Autodesk Inventor part; units mm, degrees
(part 2 of 2)
sketch "Sketch5" plane through (-0.0003, -144.9621, -142.4319) normal (0, 0, -1) x (-1, 0, 0)
  line L0 (-2.9666, 137.688) -> (-2.1497, 137.688)
  line L1 (-2.1497, 137.688) -> (-2.1497, 133.7853)
  line L2 (-2.1497, 133.7853) -> (-2.9666, 133.7853)
  line L3 (-2.9666, 133.7853) -> (-2.9666, 135.2375)
  line L4 (-2.9666, 135.2375) -> (-8.328, 135.2375)
  line L5 (-8.328, 135.2375) -> (-8.328, 133.7853)
  line L6 (-8.328, 133.7853) -> (-9.0606, 133.7853)
  spline S0 degree 2 poles (-9.0606, 133.7853) (-9.0606, 134.6086) (-9.5274, 135.3866) (-10.1757, 135.4385) knots 0 0 0 1 2 2 2
  line L7 (-10.1757, 135.4385) -> (-10.1757, 136.2683)
  line L8 (-10.1757, 136.2683) -> (-2.9666, 136.2683)
  line L9 (-2.9666, 136.2683) -> (-2.9666, 137.688)
  spline S1 degree 2 poles (-8.9569, 129.9474) (-9.106, 129.7205) (-9.2291, 129.1175) (-9.2291, 128.6767) knots 0 0 0 1 2 2 2
  line L10 (-9.2291, 128.6767) -> (-9.2291, 127.62)
  line L11 (-9.2291, 127.62) -> (-6.221, 127.62)
  line L12 (-6.221, 127.62) -> (-6.221, 128.5535)
  spline S2 degree 2 poles (-6.221, 128.5535) (-6.221, 129.0138) (-6.3831, 129.7464) (-6.636, 129.9992) knots 0 0 0 1 2 2 2
  spline S3 degree 2 poles (-6.636, 129.9992) (-6.8564, 130.2326) (-7.4787, 130.453) (-7.8937, 130.453) knots 0 0 0 1 2 2 2
  spline S4 degree 2 poles (-7.8937, 130.453) (-8.2437, 130.453) (-8.7818, 130.2067) (-8.9569, 129.9474) knots 0 0 0 1 2 2 2
  line L13 (-5.6311, 129.902) -> (-2.1497, 132.748)
  line L14 (-2.1497, 132.748) -> (-2.1497, 131.3671)
  line L15 (-2.1497, 131.3671) -> (-5.3329, 128.8388)
  line L16 (-5.3329, 128.8388) -> (-5.3329, 127.62)
  line L17 (-5.3329, 127.62) -> (-2.1497, 127.62)
  line L18 (-2.1497, 127.62) -> (-2.1497, 126.5568)
  line L19 (-2.1497, 126.5568) -> (-10.1497, 126.5568)
  line L20 (-10.1497, 126.5568) -> (-10.1497, 128.6184)
  spline S5 degree 2 poles (-10.1497, 128.6184) (-10.1497, 129.3056) (-10.0006, 130.2326) (-9.7283, 130.654) knots 0 0 0 1 2 2 2
  spline S6 degree 2 poles (-9.7283, 130.654) (-9.4561, 131.0754) (-8.6068, 131.5616) (-7.9779, 131.5616) knots 0 0 0 1 2 2 2
  spline S7 degree 2 poles (-7.9779, 131.5616) (-7.1027, 131.5616) (-5.9163, 130.667) (-5.6311, 129.902) knots 0 0 0 1 2 2 2
  circle A0 centre (-58.0001, 28.9999) radius 15
  circle A1 centre (-58.0001, 28.9999) radius 17.5
  circle A2 centre (-58.0002, 115.962) radius 15
  circle A3 centre (-58.0002, 115.962) radius 17.5
  spline S8 degree 2 poles (-53.3136, 62.2242) (-52.7949, 62.2242) (-52.017, 61.9487) (-51.7414, 61.6569) knots 0 0 0 1 2 2 2
  spline S9 degree 2 poles (-51.7414, 61.6569) (-51.4254, 61.3409) (-51.2228, 60.4252) (-51.2228, 59.8498) knots 0 0 0 1 2 2 2
  line L21 (-51.2228, 59.8498) -> (-51.2228, 58.6829)
  line L22 (-51.2228, 58.6829) -> (-54.9829, 58.6829)
  line L23 (-54.9829, 58.6829) -> (-54.9829, 60.0038)
  spline S10 degree 2 poles (-54.9829, 60.0038) (-54.9829, 60.5548) (-54.829, 61.3085) (-54.6426, 61.5921) knots 0 0 0 1 2 2 2
  spline S11 degree 2 poles (-54.6426, 61.5921) (-54.4238, 61.9163) (-53.7512, 62.2242) (-53.3136, 62.2242) knots 0 0 0 1 2 2 2
  spline S12 degree 2 poles (-55.6069, 62.4754) (-55.9473, 61.9487) (-56.1337, 60.7898) (-56.1337, 59.9308) knots 0 0 0 1 2 2 2
  line L24 (-56.1337, 59.9308) -> (-56.1337, 57.3539)
  line L25 (-56.1337, 57.3539) -> (-46.1337, 57.3539)
  line L26 (-46.1337, 57.3539) -> (-46.1337, 58.6829)
  line L27 (-46.1337, 58.6829) -> (-50.1126, 58.6829)
  line L28 (-50.1126, 58.6829) -> (-50.1126, 60.2064)
  line L29 (-50.1126, 60.2064) -> (-46.1337, 63.3668)
  line L30 (-46.1337, 63.3668) -> (-46.1337, 65.0929)
  line L31 (-46.1337, 65.0929) -> (-50.4854, 61.5354)
  spline S13 degree 2 poles (-50.4854, 61.5354) (-50.8419, 62.4916) (-52.3249, 63.6099) (-53.4189, 63.6099) knots 0 0 0 1 2 2 2
  spline S14 degree 2 poles (-53.4189, 63.6099) (-54.205, 63.6099) (-55.2666, 63.0022) (-55.6069, 62.4754) knots 0 0 0 1 2 2 2
  spline S15 degree 2 poles (-38.2398, 60.268) (-36.6644, 60.268) (-34.9918, 58.952) (-34.9918, 57.8434) knots 0 0 0 1 2 2 2
  spline S16 degree 2 poles (-34.9918, 57.8434) (-34.9918, 56.7348) (-36.6644, 55.4122) (-38.2398, 55.4122) knots 0 0 0 1 2 2 2
  spline S17 degree 2 poles (-38.2398, 55.4122) (-39.0177, 55.4122) (-40.2495, 55.7494) (-40.6579, 56.067) knots 0 0 0 1 2 2 2
  spline S18 degree 2 poles (-40.6579, 56.067) (-41.0858, 56.3977) (-41.4878, 57.2664) (-41.4878, 57.8434) knots 0 0 0 1 2 2 2
  spline S19 degree 2 poles (-41.4878, 57.8434) (-41.4878, 58.4009) (-41.0728, 59.2956) (-40.6579, 59.6132) knots 0 0 0 1 2 2 2
  spline S20 degree 2 poles (-40.6579, 59.6132) (-40.256, 59.9244) (-39.0307, 60.268) (-38.2398, 60.268) knots 0 0 0 1 2 2 2
  spline S21 degree 2 poles (-38.2398, 54.3037) (-37.2544, 54.3037) (-35.692, 54.7964) (-35.1604, 55.2567) knots 0 0 0 1 2 2 2
  spline S22 degree 2 poles (-35.1604, 55.2567) (-34.6223, 55.7299) (-34.0712, 57.0265) (-34.0712, 57.8369) knots 0 0 0 1 2 2 2
  spline S23 degree 2 poles (-34.0712, 57.8369) (-34.0712, 58.6213) (-34.6028, 59.9244) (-35.1604, 60.4171) knots 0 0 0 1 2 2 2
  spline S24 degree 2 poles (-35.1604, 60.4171) (-35.692, 60.8839) (-37.2673, 61.3766) (-38.2398, 61.3766) knots 0 0 0 1 2 2 2
  spline S25 degree 2 poles (-38.2398, 61.3766) (-39.2382, 61.3766) (-40.7941, 60.8709) (-41.3257, 60.4171) knots 0 0 0 1 2 2 2
  spline S26 degree 2 poles (-41.3257, 60.4171) (-41.8378, 59.9633) (-42.4083, 58.6537) (-42.4083, 57.8369) knots 0 0 0 1 2 2 2
  spline S27 degree 2 poles (-42.4083, 57.8369) (-42.4083, 57.033) (-41.8573, 55.7299) (-41.3257, 55.2631) knots 0 0 0 1 2 2 2
  spline S28 degree 2 poles (-41.3257, 55.2631) (-40.7746, 54.8028) (-39.2446, 54.3037) (-38.2398, 54.3037) knots 0 0 0 1 2 2 2
  line L32 (-35.1863, 82.7186) -> (-38.1555, 82.7186)
  line L33 (-38.1555, 82.7186) -> (-38.1555, 86.3944)
  line L34 (-38.1555, 86.3944) -> (-39.102, 86.3944)
  line L35 (-39.102, 86.3944) -> (-39.102, 82.7186)
  line L36 (-39.102, 82.7186) -> (-41.2933, 82.7186)
  line L37 (-41.2933, 82.7186) -> (-41.2933, 86.6602)
  line L38 (-41.2933, 86.6602) -> (-42.2398, 86.6602)
  line L39 (-42.2398, 86.6602) -> (-42.2398, 81.6554)
  line L40 (-42.2398, 81.6554) -> (-34.2398, 81.6554)
  line L41 (-34.2398, 81.6554) -> (-34.2398, 86.6602)
  line L42 (-34.2398, 86.6602) -> (-35.1863, 86.6602)
  line L43 (-35.1863, 86.6602) -> (-35.1863, 82.7186)
  line L44 (-42.2398, 77.2469) -> (-42.2398, 76.1837)
  line L45 (-42.2398, 76.1837) -> (-34.2398, 76.1837)
  line L46 (-34.2398, 76.1837) -> (-34.2398, 80.8191)
  line L47 (-34.2398, 80.8191) -> (-35.1863, 80.8191)
  line L48 (-35.1863, 80.8191) -> (-35.1863, 77.2469)
  line L49 (-35.1863, 77.2469) -> (-42.2398, 77.2469)
  spline S29 degree 2 poles (-25.1959, 17.9986) (-24.6221, 17.9986) (-23.7761, 17.6777) (-23.4163, 17.3179) knots 0 0 0 1 2 2 2
  spline S30 degree 2 poles (-23.4163, 17.3179) (-23.0079, 16.9289) (-22.6967, 15.7328) (-22.6967, 14.7604) knots 0 0 0 1 2 2 2
  line L50 (-22.6967, 14.7604) -> (-22.6967, 13.6712)
  line L51 (-22.6967, 13.6712) -> (-27.4811, 13.6712)
  line L52 (-27.4811, 13.6712) -> (-27.4811, 14.9938)
  spline S31 degree 2 poles (-27.4811, 14.9938) (-27.4811, 15.7425) (-27.2769, 16.7539) (-27.0241, 17.1331) knots 0 0 0 1 2 2 2
  spline S32 degree 2 poles (-27.0241, 17.1331) (-26.7323, 17.5707) (-25.8182, 17.9986) (-25.1959, 17.9986) knots 0 0 0 1 2 2 2
  line L53 (-28.862, 12.0764) -> (-16.862, 12.0764)
  line L54 (-16.862, 12.0764) -> (-16.862, 13.6712)
  line L55 (-16.862, 13.6712) -> (-21.3352, 13.6712)
  line L56 (-21.3352, 13.6712) -> (-21.3352, 15.0229)
  spline S33 degree 2 poles (-21.3352, 15.0229) (-21.3352, 16.3066) (-21.9673, 17.9889) (-22.58, 18.6113) knots 0 0 0 1 2 2 2
  spline S34 degree 2 poles (-22.58, 18.6113) (-23.0662, 19.1072) (-24.4665, 19.6615) (-25.2445, 19.6615) knots 0 0 0 1 2 2 2
  spline S35 degree 2 poles (-25.2445, 19.6615) (-26.2461, 19.6615) (-27.6561, 18.903) (-28.1132, 18.232) knots 0 0 0 1 2 2 2
  spline S36 degree 2 poles (-28.1132, 18.232) (-28.5119, 17.6583) (-28.862, 16.1607) (-28.862, 15.091) knots 0 0 0 1 2 2 2
  line L57 (-28.862, 15.091) -> (-28.862, 12.0764)
  line L58 (-10.1757, 136.2683) -> (-10.1757, 135.4385)
  spline S37 degree 2 poles (-10.1757, 135.4385) (-9.5274, 135.3866) (-9.0606, 134.6086) (-9.0606, 133.7853) knots 0 0 0 1 2 2 2
  line L59 (-9.0606, 133.7853) -> (-8.328, 133.7853)
  line L60 (-8.328, 133.7853) -> (-8.328, 135.2375)
  line L61 (-8.328, 135.2375) -> (-2.9666, 135.2375)
  line L62 (-2.9666, 135.2375) -> (-2.9666, 133.7853)
  line L63 (-2.9666, 133.7853) -> (-2.1497, 133.7853)
  line L64 (-2.1497, 133.7853) -> (-2.1497, 137.688)
  line L65 (-2.1497, 137.688) -> (-2.9666, 137.688)
  line L66 (-2.9666, 137.688) -> (-2.9666, 136.2683)
  line L67 (-2.9666, 136.2683) -> (-10.1757, 136.2683)
  line L68 (-46.0033, 82.349) -> (-46.0033, 83.678)
  line L69 (-46.0033, 83.678) -> (-50.8169, 83.678)
  line L70 (-50.8169, 83.678) -> (-50.8169, 88.135)
  line L71 (-50.8169, 88.135) -> (-52, 88.135)
  line L72 (-52, 88.135) -> (-52, 83.678)
  line L73 (-52, 83.678) -> (-54.8201, 83.678)
  line L74 (-54.8201, 83.678) -> (-54.8201, 88.3295)
  line L75 (-54.8201, 88.3295) -> (-56.0033, 88.3295)
  line L76 (-56.0033, 88.3295) -> (-56.0033, 82.349)
  line L77 (-56.0033, 82.349) -> (-46.0033, 82.349)
  line L78 (-42.2398, 68.2356) -> (-42.2398, 67.1724)
  line L79 (-42.2398, 67.1724) -> (-37.222, 67.1724)
  spline S38 degree 2 poles (-37.222, 67.1724) (-36.6839, 67.1724) (-35.9383, 67.0298) (-35.6336, 66.8288) knots 0 0 0 1 2 2 2
  spline S39 degree 2 poles (-35.6336, 66.8288) (-35.3095, 66.6148) (-34.9788, 65.8369) (-34.9788, 65.3377) knots 0 0 0 1 2 2 2
  spline S40 degree 2 poles (-34.9788, 65.3377) (-34.9788, 64.8061) (-35.3095, 64.067) (-35.6336, 63.8531) knots 0 0 0 1 2 2 2
  spline S41 degree 2 poles (-35.6336, 63.8531) (-35.9383, 63.6521) (-36.6904, 63.5095) (-37.2479, 63.5095) knots 0 0 0 1 2 2 2
  line L80 (-37.2479, 63.5095) -> (-42.2398, 63.5095)
  line L81 (-42.2398, 63.5095) -> (-42.2398, 62.4463)
  line L82 (-42.2398, 62.4463) -> (-37.2479, 62.4463)
  spline S42 degree 2 poles (-37.2479, 62.4463) (-36.3921, 62.4463) (-35.2252, 62.7899) (-34.8103, 63.2113) knots 0 0 0 1 2 2 2
  spline S43 degree 2 poles (-34.8103, 63.2113) (-34.4408, 63.5808) (-34.0712, 64.631) (-34.0712, 65.3377) knots 0 0 0 1 2 2 2
  spline S44 degree 2 poles (-34.0712, 65.3377) (-34.0712, 66.0768) (-34.4343, 67.0881) (-34.8103, 67.4706) knots 0 0 0 1 2 2 2
  spline S45 degree 2 poles (-34.8103, 67.4706) (-35.2187, 67.8985) (-36.4116, 68.2356) (-37.2479, 68.2356) knots 0 0 0 1 2 2 2
  line L83 (-37.2479, 68.2356) -> (-42.2398, 68.2356)
  line L84 (-41.2933, 93.4414) -> (-42.2398, 93.4414)
  line L85 (-42.2398, 93.4414) -> (-42.2398, 87.0103)
  line L86 (-42.2398, 87.0103) -> (-41.2933, 87.0103)
  line L87 (-41.2933, 87.0103) -> (-41.2933, 89.6943)
  line L88 (-41.2933, 89.6943) -> (-34.2398, 89.6943)
  line L89 (-34.2398, 89.6943) -> (-34.2398, 90.7575)
  line L90 (-34.2398, 90.7575) -> (-41.2933, 90.7575)
  line L91 (-41.2933, 90.7575) -> (-41.2933, 93.4414)
  line L92 (-41.2933, 75.3733) -> (-42.2398, 75.3733)
  line L93 (-42.2398, 75.3733) -> (-42.2398, 68.9422)
  line L94 (-42.2398, 68.9422) -> (-41.2933, 68.9422)
  line L95 (-41.2933, 68.9422) -> (-41.2933, 71.6262)
  line L96 (-41.2933, 71.6262) -> (-34.2398, 71.6262)
  line L97 (-34.2398, 71.6262) -> (-34.2398, 72.6894)
  line L98 (-34.2398, 72.6894) -> (-41.2933, 72.6894)
  line L99 (-41.2933, 72.6894) -> (-41.2933, 75.3733)
  line L100 (-19.5848, 29.5999) -> (-19.5848, 29.4832)
  spline S46 degree 2 poles (-19.5848, 29.4832) (-19.4001, 29.2985) (-18.8749, 28.6469) (-18.6221, 28.2093) knots 0 0 0 1 2 2 2
  spline S47 degree 2 poles (-18.6221, 28.2093) (-18.3693, 27.7523) (-18.0289, 26.5756) (-18.0289, 25.8852) knots 0 0 0 1 2 2 2
  spline S48 degree 2 poles (-18.0289, 25.8852) (-18.0289, 25.1267) (-18.6318, 23.775) (-19.225, 23.2693) knots 0 0 0 1 2 2 2
  spline S49 degree 2 poles (-19.225, 23.2693) (-19.8377, 22.7539) (-21.6173, 22.1607) (-22.8523, 22.1607) knots 0 0 0 1 2 2 2
  spline S50 degree 2 poles (-22.8523, 22.1607) (-24.0095, 22.1607) (-25.8668, 22.7247) (-26.4795, 23.2304) knots 0 0 0 1 2 2 2
  spline S51 degree 2 poles (-26.4795, 23.2304) (-27.0824, 23.7458) (-27.7145, 25.1169) (-27.7145, 25.8852) knots 0 0 0 1 2 2 2
  spline S52 degree 2 poles (-27.7145, 25.8852) (-27.7145, 26.5853) (-27.3936, 27.6647) (-27.1408, 28.1218) knots 0 0 0 1 2 2 2
  spline S53 degree 2 poles (-27.1408, 28.1218) (-26.8782, 28.5983) (-26.3336, 29.2596) (-26.1391, 29.4735) knots 0 0 0 1 2 2 2
  line L101 (-26.1391, 29.4735) -> (-26.1391, 29.5999)
  line L102 (-26.1391, 29.5999) -> (-28.0646, 29.5999)
  spline S54 degree 2 poles (-28.0646, 29.5999) (-28.2785, 29.2012) (-28.6383, 28.3941) (-28.7647, 28.0051) knots 0 0 0 1 2 2 2
  spline S55 degree 2 poles (-28.7647, 28.0051) (-28.9009, 27.5578) (-29.0759, 26.4978) (-29.0759, 25.8949) knots 0 0 0 1 2 2 2
  spline S56 degree 2 poles (-29.0759, 25.8949) (-29.0759, 24.6793) (-28.2299, 22.715) (-27.4228, 21.9954) knots 0 0 0 1 2 2 2
  spline S57 degree 2 poles (-27.4228, 21.9954) (-26.5962, 21.266) (-24.3596, 20.4978) (-22.8523, 20.4978) knots 0 0 0 1 2 2 2
  spline S58 degree 2 poles (-22.8523, 20.4978) (-21.3352, 20.4978) (-19.0014, 21.2855) (-18.2234, 22.0051) knots 0 0 0 1 2 2 2
  spline S59 degree 2 poles (-18.2234, 22.0051) (-17.4357, 22.7247) (-16.648, 24.6988) (-16.648, 25.8657) knots 0 0 0 1 2 2 2
  spline S60 degree 2 poles (-16.648, 25.8657) (-16.648, 26.5853) (-16.8231, 27.48) (-16.9981, 28.0051) knots 0 0 0 1 2 2 2
  spline S61 degree 2 poles (-16.9981, 28.0051) (-17.1537, 28.501) (-17.4941, 29.2012) (-17.6788, 29.5999) knots 0 0 0 1 2 2 2
  line L103 (-17.6788, 29.5999) -> (-19.5848, 29.5999)
  spline S62 degree 2 poles (-7.8937, 130.453) (-7.4787, 130.453) (-6.8564, 130.2326) (-6.636, 129.9992) knots 0 0 0 1 2 2 2
  spline S63 degree 2 poles (-6.636, 129.9992) (-6.3831, 129.7464) (-6.221, 129.0138) (-6.221, 128.5535) knots 0 0 0 1 2 2 2
  line L104 (-6.221, 128.5535) -> (-6.221, 127.62)
  line L105 (-6.221, 127.62) -> (-9.2291, 127.62)
  line L106 (-9.2291, 127.62) -> (-9.2291, 128.6767)
  spline S64 degree 2 poles (-9.2291, 128.6767) (-9.2291, 129.1175) (-9.106, 129.7205) (-8.9569, 129.9474) knots 0 0 0 1 2 2 2
  spline S65 degree 2 poles (-8.9569, 129.9474) (-8.7818, 130.2067) (-8.2437, 130.453) (-7.8937, 130.453) knots 0 0 0 1 2 2 2
  spline S66 degree 2 poles (-9.7283, 130.654) (-10.0006, 130.2326) (-10.1497, 129.3056) (-10.1497, 128.6184) knots 0 0 0 1 2 2 2
  line L107 (-10.1497, 128.6184) -> (-10.1497, 126.5568)
  line L108 (-10.1497, 126.5568) -> (-2.1497, 126.5568)
  line L109 (-2.1497, 126.5568) -> (-2.1497, 127.62)
  line L110 (-2.1497, 127.62) -> (-5.3329, 127.62)
  line L111 (-5.3329, 127.62) -> (-5.3329, 128.8388)
  line L112 (-5.3329, 128.8388) -> (-2.1497, 131.3671)
  line L113 (-2.1497, 131.3671) -> (-2.1497, 132.748)
  line L114 (-2.1497, 132.748) -> (-5.6311, 129.902)
  spline S67 degree 2 poles (-5.6311, 129.902) (-5.9163, 130.667) (-7.1027, 131.5616) (-7.9779, 131.5616) knots 0 0 0 1 2 2 2
  spline S68 degree 2 poles (-7.9779, 131.5616) (-8.6068, 131.5616) (-9.4561, 131.0754) (-9.7283, 130.654) knots 0 0 0 1 2 2 2
  line L115 (-80, 1.9999) -> (3, 2)
  line L116 (2.9997, 142.9621) -> (3, 2)
  line L117 (2.9997, 142.9621) -> (-80.0003, 142.9619)
  line L118 (-80, 1.9999) -> (-80.0003, 142.9619)
  circle A4 centre (-65.2412, 59.9999) radius 3.35
  circle A5 centre (-65.2412, 84.962) radius 3.35
  line L119 (-14.0356, 12.0349) -> (-4.0356, 12.0349)
  line L120 (-4.0356, 12.0349) -> (-4.0357, 29.0349)
  line L121 (-4.0357, 29.0349) -> (-14.0357, 29.0349)
  line L122 (-14.0357, 29.0349) -> (-14.0356, 12.0349)
  line L123 (-63.526, 17.7389) -> (-63.526, 41.2748) construction
  line L124 (-63.526, 41.2748) -> (-53.9143, 41.2748) construction
  line L125 (-53.9143, 41.2748) -> (-53.9143, 17.7389) construction
  line L126 (-53.9143, 17.7389) -> (-63.526, 17.7389) construction
  line L127 (-63.308, 105.7482) -> (-63.308, 126.3521) construction
  line L128 (-63.308, 126.3521) -> (-53.7172, 126.3521) construction
  line L129 (-53.7172, 126.3521) -> (-53.7172, 105.7482) construction
  line L130 (-53.7172, 105.7482) -> (-63.308, 105.7482) construction
  spline S69 degree 2 poles (-57.7913, 18.1574) (-59.5954, 18.1574) (-60.4666, 19.1657) knots 0 0 0 1 1 1
  spline S70 degree 2 poles (-60.4666, 19.1657) (-61.1937, 20.0026) (-61.1937, 21.2099) knots 0 0 0 1 1 1
  spline S71 degree 2 poles (-61.1937, 21.2099) (-61.1937, 22.5545) (-59.4308, 24.2625) (-57.8805, 24.2625) knots 0 0 0 1 2 2 2
  spline S72 degree 2 poles (-57.8805, 24.2625) (-56.6251, 24.2625) (-55.1777, 23.508) (-54.382, 22.0674) (-54.382, 21.2099) knots 0 0 0 1 2 3 3 3
  spline S73 degree 2 poles (-54.382, 21.2099) (-54.382, 19.8449) (-56.1381, 18.1574) (-57.7913, 18.1574) knots 0 0 0 1 2 2 2
  spline S74 degree 2 poles (-57.7844, 19.2961) (-56.536, 19.2961) (-55.2875, 20.3868) (-55.2875, 21.2099) knots 0 0 0 1 2 2 2
  spline S75 degree 2 poles (-55.2875, 21.2099) (-55.2875, 22.0331) (-56.5428, 23.1238) (-57.8256, 23.1238) knots 0 0 0 1 2 2 2
  spline S76 degree 2 poles (-57.8256, 23.1238) (-59.0329, 23.1238) (-60.2814, 22.0263) (-60.2814, 21.2099) knots 0 0 0 1 2 2 2
  spline S77 degree 2 poles (-60.2814, 21.2099) (-60.2814, 20.3868) (-59.0398, 19.2961) (-57.7844, 19.2961) knots 0 0 0 1 2 2 2
  line L131 (-56.4742, 25.1131) -> (-56.6457, 26.2038)
  spline S78 degree 2 poles (-56.6457, 26.2038) (-55.9872, 26.293) (-55.2875, 27.1368) (-55.2875, 27.8982) knots 0 0 0 1 2 2 2
  spline S79 degree 2 poles (-55.2875, 27.8982) (-55.2875, 28.6596) (-55.9117, 29.4005) (-56.3302, 29.4005) knots 0 0 0 1 2 2 2
  spline S80 degree 2 poles (-56.3302, 29.4005) (-56.7006, 29.4005) (-56.9201, 29.0712) knots 0 0 0 1 1 1
  spline S81 degree 2 poles (-56.9201, 29.0712) (-57.0642, 28.8448) (-57.2905, 27.9394) knots 0 0 0 1 1 1
  spline S82 degree 2 poles (-57.2905, 27.9394) (-57.5992, 26.7252) (-58.0451, 25.7854) (-58.8408, 25.2984) (-59.3142, 25.2984) knots 0 0 0 1 2 3 3 3
  spline S83 degree 2 poles (-59.3142, 25.2984) (-59.7532, 25.2984) (-60.494, 25.6962) (-60.741, 26.0392) knots 0 0 0 1 2 2 2
  spline S84 degree 2 poles (-60.741, 26.0392) (-60.9331, 26.2999) (-61.1937, 27.1916) (-61.1937, 27.7061) knots 0 0 0 1 2 2 2
  spline S85 degree 2 poles (-61.1937, 27.7061) (-61.1937, 28.4744) (-60.7478, 29.6337) (-59.9933, 30.1894) (-59.3622, 30.2923) knots 0 0 0 1 2 3 3 3
  line L132 (-59.3622, 30.2923) -> (-59.2181, 29.2084)
  spline S86 degree 2 poles (-59.2181, 29.2084) (-59.7257, 29.133) (-60.2882, 28.4264) (-60.2882, 27.7816) knots 0 0 0 1 2 2 2
  spline S87 degree 2 poles (-60.2882, 27.7816) (-60.2882, 27.0202) (-59.7806, 26.3685) (-59.4445, 26.3685) knots 0 0 0 1 2 2 2
  spline S88 degree 2 poles (-59.4445, 26.3685) (-59.2318, 26.3685) (-59.0603, 26.5057) knots 0 0 0 1 1 1
  spline S89 degree 2 poles (-59.0603, 26.5057) (-58.882, 26.636) (-58.7654, 26.931) knots 0 0 0 1 1 1
  spline S90 degree 2 poles (-58.7654, 26.931) (-58.7036, 27.0956) (-58.4773, 27.9051) knots 0 0 0 1 1 1
  spline S91 degree 2 poles (-58.4773, 27.9051) (-58.1686, 29.0781) (-57.7707, 30.011) (-57.0093, 30.5392) (-56.4399, 30.5392) knots 0 0 0 1 2 3 3 3
  spline S92 degree 2 poles (-56.4399, 30.5392) (-55.8911, 30.5392) (-54.9171, 29.8944) (-54.382, 28.6734) (-54.382, 27.9051) knots 0 0 0 1 2 3 3 3
  spline S93 degree 2 poles (-54.382, 27.9051) (-54.382, 26.636) (-55.4384, 25.2984) (-56.4742, 25.1131) knots 0 0 0 1 2 2 2
  line L133 (-54.526, 36.1162) -> (-55.4864, 36.1162)
  spline S94 degree 2 poles (-55.4864, 36.1162) (-54.382, 35.3548) (-54.382, 34.0514) knots 0 0 0 1 1 1
  spline S95 degree 2 poles (-54.382, 34.0514) (-54.382, 33.4752) (-54.821, 32.4737) (-55.4933, 31.9866) (-55.9803, 31.8906) knots 0 0 0 1 2 3 3 3
  spline S96 degree 2 poles (-55.9803, 31.8906) (-56.3027, 31.822) (-57.0093, 31.822) knots 0 0 0 1 1 1
  line L134 (-57.0093, 31.822) -> (-61.0497, 31.822)
  line L135 (-61.0497, 31.822) -> (-61.0497, 32.9264)
  line L136 (-61.0497, 32.9264) -> (-57.4346, 32.9264)
  spline S97 degree 2 poles (-57.4346, 32.9264) (-56.5703, 32.9264) (-56.2684, 32.995) knots 0 0 0 1 1 1
  spline S98 degree 2 poles (-56.2684, 32.995) (-55.8294, 33.0979) (-55.3355, 33.7702) (-55.3355, 34.2709) knots 0 0 0 1 2 2 2
  spline S99 degree 2 poles (-55.3355, 34.2709) (-55.3355, 34.7648) (-55.8431, 35.636) (-56.7212, 35.9996) (-57.5581, 35.9996) knots 0 0 0 1 2 3 3 3
  line L137 (-57.5581, 35.9996) -> (-61.0497, 35.9996)
  line L138 (-61.0497, 35.9996) -> (-61.0497, 37.104)
  line L139 (-61.0497, 37.104) -> (-54.526, 37.104)
  line L140 (-54.526, 37.104) -> (-54.526, 36.1162)
  line L141 (-56.7555, 39.4295) -> (-61.5299, 39.0933)
  line L142 (-61.5299, 39.0933) -> (-63.526, 39.0933)
  line L143 (-63.526, 39.0933) -> (-63.526, 40.4653)
  line L144 (-63.526, 40.4653) -> (-61.5299, 40.4653)
  line L145 (-61.5299, 40.4653) -> (-56.7555, 40.1429)
  line L146 (-56.7555, 40.1429) -> (-56.7555, 39.4295)
  line L147 (-54.526, 39.1413) -> (-55.7814, 39.1413)
  line L148 (-55.7814, 39.1413) -> (-55.7814, 40.4173)
  line L149 (-55.7814, 40.4173) -> (-54.526, 40.4173)
  line L150 (-54.526, 40.4173) -> (-54.526, 39.1413)
  spline S100 degree 2 poles (-56.1932, 112.507) (-55.886, 112.507) (-55.1878, 112.1369) (-54.5524, 111.3828) (-54.1684, 110.2378) (-54.1684, 109.5186) knots 0 0 0 1 2 3 4 4 4
  spline S101 degree 2 poles (-54.1684, 109.5186) (-54.1684, 107.9965) (-55.9488, 106.2789) (-57.443, 106.2789) knots 0 0 0 1 2 2 2
  spline S102 degree 2 poles (-57.443, 106.2789) (-58.4554, 106.2789) (-60.0124, 107.0609) (-60.8643, 108.5481) (-60.8643, 109.5814) knots 0 0 0 1 2 3 3 3
  spline S103 degree 2 poles (-60.8643, 109.5814) (-60.8643, 110.2238) (-60.4872, 111.2921) (-59.9007, 112.0322) (-59.2304, 112.4232) (-58.9442, 112.4232) knots 0 0 0 1 2 3 4 4 4
  spline S104 degree 2 poles (-58.9442, 112.4232) (-58.6439, 112.4232) (-58.232, 111.9833) (-58.232, 111.6691) knots 0 0 0 1 2 2 2
  spline S105 degree 2 poles (-58.232, 111.6691) (-58.232, 111.4666) (-58.4484, 111.1943) (-58.6858, 111.0268) knots 0 0 0 1 2 2 2
  spline S106 degree 2 poles (-58.6858, 111.0268) (-59.1397, 110.7195) (-59.6005, 110.0632) (-59.6005, 109.5535) knots 0 0 0 1 2 2 2
  spline S107 degree 2 poles (-59.6005, 109.5535) (-59.6005, 108.8274) (-58.4554, 107.9337) (-57.4709, 107.9337) knots 0 0 0 1 2 2 2
  spline S108 degree 2 poles (-57.4709, 107.9337) (-57.0031, 107.9337) (-56.2211, 108.1641) (-55.6765, 108.597) (-55.3902, 109.2114) (-55.3902, 109.5814) knots 0 0 0 1 2 3 4 4 4
  spline S109 degree 2 poles (-55.3902, 109.5814) (-55.3902, 110.0772) (-55.8511, 110.7824) (-56.3189, 111.0547) knots 0 0 0 1 2 2 2
  spline S110 degree 2 poles (-56.3189, 111.0547) (-56.5982, 111.2013) (-56.9124, 111.5574) (-56.9124, 111.8088) knots 0 0 0 1 2 2 2
  spline S111 degree 2 poles (-56.9124, 111.8088) (-56.9124, 112.109) (-56.4515, 112.507) (-56.1932, 112.507) knots 0 0 0 1 2 2 2
  line L151 (-62.3654, 115.4674) -> (-59.8449, 115.4674)
  spline S112 degree 2 poles (-59.8449, 115.4674) (-60.3266, 115.9352) (-60.8433, 116.8987) (-60.8433, 117.6109) knots 0 0 0 1 2 2 2
  spline S113 degree 2 poles (-60.8433, 117.6109) (-60.8433, 118.4278) (-60.0613, 119.6637) (-58.5881, 120.3479) (-57.5687, 120.3479) knots 0 0 0 1 2 3 3 3
  spline S114 degree 2 poles (-57.5687, 120.3479) (-56.8216, 120.3479) (-55.5718, 119.9709) (-54.6571, 119.2447) (-54.1544, 118.2114) (-54.1544, 117.59) knots 0 0 0 1 2 3 4 4 4
  spline S115 degree 2 poles (-54.1544, 117.59) (-54.1544, 117.2129) (-54.3359, 116.5427) (-54.6292, 116.0679) (-54.9434, 115.7397) (-55.2576, 115.4674) knots 0 0 0 1 2 3 4 4 4
  line L152 (-55.2576, 115.4674) -> (-55.097, 115.4674)
  spline S116 degree 2 poles (-55.097, 115.4674) (-54.6292, 115.4674) (-54.1544, 115.0205) (-54.1544, 114.6784) knots 0 0 0 1 2 2 2
  spline S117 degree 2 poles (-54.1544, 114.6784) (-54.1544, 114.3293) (-54.6292, 113.9104) (-55.097, 113.9104) knots 0 0 0 1 2 2 2
  line L153 (-55.097, 113.9104) -> (-62.2956, 113.9104)
  spline S118 degree 2 poles (-62.2956, 113.9104) (-62.7983, 113.9104) (-63.308, 114.3153) (-63.308, 114.6784) knots 0 0 0 1 2 2 2
  spline S119 degree 2 poles (-63.308, 114.6784) (-63.308, 115.0555) (-62.8193, 115.4674) (-62.3654, 115.4674) knots 0 0 0 1 2 2 2
  spline S120 degree 2 poles (-57.4639, 115.5442) (-56.4795, 115.5442) (-55.4252, 116.4449) (-55.4252, 117.171) knots 0 0 0 1 2 2 2
  spline S121 degree 2 poles (-55.4252, 117.171) (-55.4252, 117.7925) (-56.5074, 118.6932) (-57.5128, 118.6932) knots 0 0 0 1 2 2 2
  spline S122 degree 2 poles (-57.5128, 118.6932) (-58.1691, 118.6932) (-59.1117, 118.3161) (-59.6214, 117.6319) (-59.6214, 117.171) knots 0 0 0 1 2 3 3 3
  spline S123 degree 2 poles (-59.6214, 117.171) (-59.6214, 116.7032) (-59.1117, 115.9701) (-58.1342, 115.5442) (-57.4639, 115.5442) knots 0 0 0 1 2 3 3 3
  line L154 (-60.7106, 121.7583) -> (-60.7106, 121.9399)
  line L155 (-60.7106, 121.9399) -> (-61.7021, 121.9399)
  spline S124 degree 2 poles (-61.7021, 121.9399) (-62.1001, 121.9399) (-62.547, 121.9818) (-62.7145, 122.0795) knots 0 0 0 1 2 2 2
  spline S125 degree 2 poles (-62.7145, 122.0795) (-62.8821, 122.1773) (-63.0916, 122.5403) (-63.0916, 122.7638) knots 0 0 0 1 2 2 2
  spline S126 degree 2 poles (-63.0916, 122.7638) (-63.0916, 123.078) (-62.8542, 123.3293) knots 0 0 0 1 1 1
  spline S127 degree 2 poles (-62.8542, 123.3293) (-62.7006, 123.4969) (-62.2467, 123.5877) (-61.8348, 123.5877) knots 0 0 0 1 2 2 2
  line L156 (-61.8348, 123.5877) -> (-60.7106, 123.5877)
  line L157 (-60.7106, 123.5877) -> (-60.7106, 124.1881)
  spline S128 degree 2 poles (-60.7106, 124.1881) (-60.7106, 124.5442) (-60.3825, 124.9073) (-60.1172, 124.9073) knots 0 0 0 1 2 2 2
  spline S129 degree 2 poles (-60.1172, 124.9073) (-59.789, 124.9073) (-59.5237, 124.3836) (-59.5237, 123.8949) knots 0 0 0 1 2 2 2
  line L158 (-59.5237, 123.8949) -> (-59.5237, 123.5877)
  line L159 (-59.5237, 123.5877) -> (-56.4864, 123.5877)
  spline S130 degree 2 poles (-56.4864, 123.5877) (-56.1024, 123.5877) (-55.6835, 123.6435) (-55.4252, 123.8739) (-55.4252, 124.1462) knots 0 0 0 1 2 3 3 3
  spline S131 degree 2 poles (-55.4252, 124.1462) (-55.4252, 124.2859) (-55.5299, 124.7816) (-55.5299, 124.9212) knots 0 0 0 1 2 2 2
  spline S132 degree 2 poles (-55.5299, 124.9212) (-55.5299, 125.1237) (-55.2087, 125.4379) (-54.9713, 125.4379) knots 0 0 0 1 2 2 2
  spline S133 degree 2 poles (-54.9713, 125.4379) (-54.5733, 125.4379) (-54.1544, 124.5721) (-54.1544, 123.7552) knots 0 0 0 1 2 2 2
  spline S134 degree 2 poles (-54.1544, 123.7552) (-54.1544, 122.9872) (-54.6711, 122.1842) (-55.5927, 121.9399) (-56.3608, 121.9399) knots 0 0 0 1 2 3 3 3
  line L160 (-56.3608, 121.9399) -> (-59.5237, 121.9399)
  line L161 (-59.5237, 121.9399) -> (-59.5237, 121.7234)
  spline S135 degree 2 poles (-59.5237, 121.7234) (-59.5237, 121.3673) (-59.8588, 120.9903) (-60.1172, 120.9903) knots 0 0 0 1 2 2 2
  spline S136 degree 2 poles (-60.1172, 120.9903) (-60.3825, 120.9903) (-60.7106, 121.3813) (-60.7106, 121.7583) knots 0 0 0 1 2 2 2
  point P0 (-0.0003, 144.9621)
  constraints: 246 end point, 59 vertical, 50 horizontal, 6 centre point, 400 other
extrude "Extrusion5" add sketch "Sketch5" against normal blind 2 contours S69 S70 S71 S72 S73 | L131 S78 S79 S80 S81 S82 S83 S84 S85 L132 S86 S87 S88 S89 S90 S91 S92 S93 | L133 S94 S95 S96 L134 L135 L136 S97 S98 S99 L137 L138 L139 L140 | L141 L142 L143 L144 L145 L146 | L147 L148 L149 L150 | S100 S101 S102 S103 S104 S105 S106 S107 S108 S109 S110 S111 | L151 S112 S113 S114 S115 L152 S116 S117 L153 S118 S119 | L154 L155 S124 S125 S126 S127 L156 L157 S128 S129 L158 L159 S130 S131 S132 S133 S134 L160 L161 S135 S136
body "Solid1"
